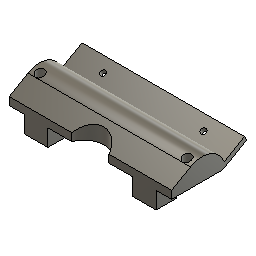
Camera Mount (Autodesk Fusion 360 design; units mm, degrees)
Autodesk Fusion 360 part; units mm, degrees
sketch "Sketch1" plane through (0, 0, 0) normal (0, 1, 0) x (1, 0, 0)
  line L0 (0, 0) -> (85, 0)
  line L1 (85, 0) -> (85, -33)
  line L2 (85, -33) -> (0, -33)
  line L3 (0, -33) -> (0, 0)
  line L4 (0, 0) -> (85, 0)
  line L5 (85, 0) -> (85, -20)
  line L6 (85, -20) -> (0, -20)
  line L7 (0, -20) -> (0, 0)
  dimension "d1" = 85
  dimension "d2" = 33
  dimension "d3" = 20
  measures "d1" distance of L0.start
  measures "d2" distance of L0.start
  measures "d3" distance of L0 L6
extrude "Extrude1" add sketch "Sketch1" along normal blind 5
extrude "Extrude2" add sketch "Sketch1" against normal blind 11 contours L1 L2 L3 L6
sketch "Sketch2" plane through (0, -11, 0) normal (0, -1, 0) x (1, 0, 0)
  line L0 (85, 20) -> (85, 33)
  line L1 (85, 33) -> (0, 33)
  line L2 (0, 33) -> (0, 20)
  line L3 (0, 20) -> (85, 20)
  line L4 (0, 33) -> (15, 33)
  line L5 (15, 33) -> (15, 20)
  line L6 (15, 20) -> (0, 20)
  line L7 (0, 20) -> (0, 33)
  line L8 (85, 33) -> (70, 33)
  line L9 (70, 33) -> (70, 20)
  line L10 (70, 20) -> (85, 20)
  line L11 (85, 20) -> (85, 33)
  dimension "d8" = 15
extrude "Extrude3" cut sketch "Sketch2" against normal blind 11 contours L1 L3 L5 L9
sketch "Sketch3" plane through (0, 5, 0) normal (0, 1, 0) x (-1, 0, 0)
  line L0 (0, 0) -> (0, 33)
  line L1 (0, 33) -> (-85, 33)
  line L2 (-85, 33) -> (-85, 0)
  line L3 (-85, 0) -> (0, 0)
  line L4 (-85, 0) -> (-95, 0)
  line L5 (-95, 0) -> (-95, 33)
  line L6 (-95, 33) -> (-85, 33)
  line L7 (-85, 33) -> (-85, 0)
  circle A0 centre (-90, 16.5) radius 2.75 construction
  line L8 (-95, 16.5) -> (-85, 16.5) construction
  line L9 (-42.5, 0) -> (-42.5, 33) construction
  line L10 (0, 0) -> (10, 0)
  line L11 (10, 0) -> (10, 33)
  line L12 (10, 33) -> (0, 33)
  line L13 (0, 33) -> (0, 0)
  circle A1 centre (5, 16.5) radius 2.75 construction
  dimension "d11" = 10
  dimension "d12" = 5.5
  measures "d11" distance of L0.start
  measures "d12" diameter of A0
extrude "Extrude4" add sketch "Sketch3" against normal blind 5 contours L0 L10 L11 L12 L13 | L2 L4 L5 L6 L7
sketch "Sketch4" plane through (-10, 0, 0) normal (-1, 0, 0) x (0, 0, 1)
  line L0 (33, 5) -> (0, 5)
  line L1 (0, 5) -> (0, 0)
  line L2 (0, 0) -> (33, 0)
  line L3 (33, 0) -> (33, 5)
  line L4 (33, 5) -> (-5.1734, 27.0394)
  line L5 (0, 5) -> (0, 0)
  line L6 (0, 0) -> (-15.5885, 9)
  line L7 (-15.5885, 9) -> (-5.1734, 27.0394)
  dimension "d17" = 30
  dimension "d50" = 18
  measures "d17" angle of L0 L4
  measures "d50" distance of L1.end
extrude "Extrude5" add sketch "Sketch4" against normal blind 105 contours L0 L1 L4 L5 L6 L7
sketch "Sketch5" plane through (95, 0, 0) normal (1, 0, 0) x (0, 0, -1)
  line L0 (-33, 5) -> (-33, 0)
  line L1 (-33, 0) -> (0, 0)
  line L2 (0, 0) -> (15.5885, 9)
  line L3 (15.5885, 9) -> (5.1734, 27.0394)
  line L4 (5.1734, 27.0394) -> (-33, 5)
  line L5 (14.0885, 11.5981) -> (5.1734, 27.0394)
  line L6 (5.1734, 27.0394) -> (-7.817, 19.5394)
  line L7 (-7.817, 19.5394) -> (1.0981, 4.0981)
  line L8 (1.0981, 4.0981) -> (14.0885, 11.5981)
  line L9 (0, 0) -> (2.5981, 1.5)
  line L10 (1.0981, 4.0981) -> (2.5981, 1.5) construction
  dimension "d48" = 3
  dimension "d51" = 3
  measures "d51" distance of L1.end
extrude "Extrude7" cut sketch "Sketch5" against normal blind 140 contours L3 L4 L5 L6 L7 L8
sketch "Sketch9" plane through (0, 2.5981, 1.5) normal (0, 0.866025, 0.5) x (1, 0, 0)
  line L0 (-10, 18) -> (-10, 3)
  line L1 (-10, 3) -> (95, 3)
  line L2 (95, 3) -> (95, 18)
  line L3 (95, 18) -> (-10, 18)
  circle A0 centre (10, 10.5) radius 1.75
  circle A1 centre (75, 10.5) radius 1.75
  dimension "d55" = 3.5
  dimension "d56" = 3.5
  dimension "d57" = 7.5
  dimension "d58" = 20
  dimension "d59" = 20
  measures "d55" diameter of A0
  measures "d56" diameter of A1
  measures "d57" distance of L3
  measures "d58" distance of L0
  measures "d59" distance of L2
extrude "Extrude11" cut sketch "Sketch9" against normal blind 16 contours A0 | A1
sketch "Sketch8" plane through (0, 0, 0) normal (0, -1, 0) x (1, 0, 0)
  line L0 (85, 20) -> (70, 20)
  line L1 (70, 20) -> (70, 33)
  line L2 (70, 33) -> (15, 33)
  line L3 (15, 33) -> (15, 20)
  line L4 (15, 20) -> (0, 20)
  line L5 (0, 20) -> (0, 33)
  line L6 (0, 33) -> (-10, 33)
  line L7 (-10, 33) -> (-10, 0)
  line L8 (95, 0) -> (95, 33)
  line L9 (95, 33) -> (85, 33)
  line L10 (85, 33) -> (85, 20)
  arc A0 (30.5, 33) -> (54.5, 33) centre (42.5, 37) ccw
  line L11 (42.5, 33) -> (54.5, 33)
  line L12 (42.5, 33) -> (30.5, 33)
  line L13 (42.5, 37) -> (42.5, 33) construction
  line L14 (-10, 0) -> (95, 0)
  dimension "d44" = 12
  dimension "d45" = 4
extrude "Extrude10" cut sketch "Sketch8" against normal blind 25 contours L2 A0 L11 L12
fillet "Fillet2" radius 15 1 edges at (42.5, 19.5394, 7.817)
sketch "Sketch10" plane through (0, 0, 0) normal (0, -1, 0) x (1, 0, 0)
  arc A0 (30.5, 33) -> (54.5, 33) centre (42.5, 37) ccw
  line L0 (30.5, 33) -> (15, 33)
  line L1 (15, 33) -> (15, 20)
  line L2 (15, 20) -> (0, 20)
  line L3 (0, 20) -> (0, 33)
  line L4 (0, 33) -> (-10, 33)
  line L5 (-10, 33) -> (-10, 0)
  line L6 (-10, 0) -> (95, 0)
  line L7 (95, 0) -> (95, 33)
  line L8 (95, 33) -> (85, 33)
  line L9 (85, 33) -> (85, 20)
  line L10 (85, 20) -> (70, 20)
  line L11 (70, 20) -> (70, 33)
  line L12 (70, 33) -> (54.5, 33)
  circle A1 centre (-5, 18) radius 2.75
  circle A2 centre (90, 18) radius 2.75
  dimension "d63" = 5.5
  dimension "d64" = 5.5
  dimension "d65" = 5
  dimension "d66" = 5
  dimension "d67" = 15
  measures "d63" diameter of A1
  measures "d64" diameter of A2
  measures "d65" distance of L5
extrude "Extrude12" cut sketch "Sketch10" against normal blind 25 contours A1 | A2
named bodies: "Camera mount 2"
